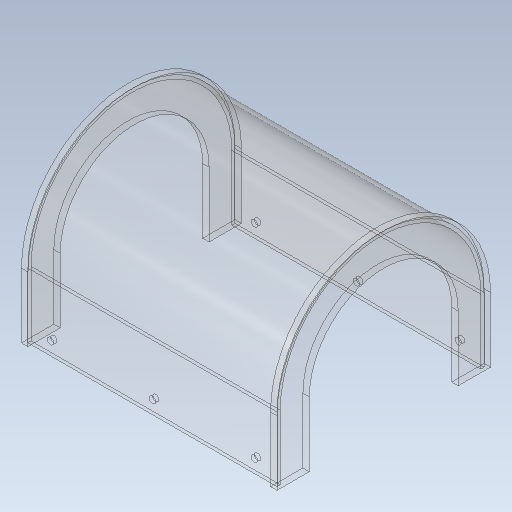
# Autodesk Inventor part: Acrilico
Saved by Autodesk Inventor 2020 (Build 240168000, 168)
## iProperties
Created: 2018-06-05
Part Number: Acrilico
Material: Plástico PMMA
Document SubType Name: Chapa
Designer: Cristiano
Density: 1.188 g/cm^3
Appearance: Policarbonato - Claro
Mass: 1478.37 g
Surface Area: 5090.38 cm^2
Volume: 1244.42 cm^3
Sheet Metal Rule: Por defecto_mm
Sheet Metal Width: 0,000 mm
Sheet Metal Length: 0,000 mm
Sheet Metal Area: 0,000 mm^2
Author: Cristiano
Autodesk Inventor part; units mm, degrees
ref_plane "YZ Plane" through (0, 0, 0) normal (1, 0, 0) x (0, 1, 0)
ref_plane "XZ Plane" through (0, 0, 0) normal (0, 1, 0) x (-1, 0, 0)
ref_plane "XY Plane" through (0, 0, 0) normal (0, 0, 1) x (1, 0, 0)
sketch "Boceto1" plane through (0, 0, 0) normal (1, 0, 0) x (0, 1, 0)
  line L0 (0, 0) -> (0, -220.3761) construction
  arc A0 (0, -155) -> (0, 155) centre (0, 0) ccw
  arc A1 (0, -160) -> (0, 160) centre (0, 0) ccw
  line L1 (0, 155) -> (0, 160) construction
  line L2 (0, -155) -> (0, -160) construction
  line L3 (0, -160) -> (-100, -160)
  line L4 (-100, -160) -> (-100, -155)
  line L5 (-100, -155) -> (0, -155)
  line L6 (0, 155) -> (-100, 155)
  line L7 (-100, 155) -> (-100, 160)
  line L8 (0, 160) -> (-100, 160)
  dimension "d1" = 155
  dimension "d4" = 160
  dimension "d7" = 100
  dimension "d8" = 5
  constraints: 18 end point, 4 point on circle, 3 collinear, 3 horizontal, 3 vertical, 2 centre point, 2 perpendicular, 1 coincident
  measures "d1" radius of A0
  measures "d4" radius of A1
  measures "d7" distance of L2.end L3.end
  measures "d8" distance of L6.end L7.end
extrude "Extrusión1" add sketch "Boceto1" along normal blind 385
sketch "Boceto2" plane through (0, -100, -160) normal (0, 0, -1) x (-1, 0, 0)
  line L0 (-385, 0) -> (-385, 100) construction
  line L1 (-385, 20) -> (0, 20) construction
  line L2 (0, 0) -> (0, 100) construction
  circle A0 centre (-350, 20) radius 5
  circle A1 centre (-192.5, 20) radius 5
  circle A2 centre (-35, 20) radius 5
  dimension "d9" = 10
  dimension "d10" = 35
  dimension "d11" = 35
  dimension "d14" = 20
  constraints: 4 point on line, 3 centre point, 2 end point, 2 equal radius, 1 midpoint, 1 perpendicular
  measures "d9" diameter of A0
  measures "d10" distance from line of L0 A0.centre
  measures "d11" distance from line of L2 A2.centre
  measures "d14" distance of L0.start L1.start
extrude "Extrusión2" cut sketch "Boceto2" against normal through all
ref_plane "Plano de trabajo1" through (192.5, 0, 0) normal (1, 0, 0) x (0, 0, -1)
sketch "Boceto3" plane through (385, 0, 0) normal (1, 0, 0) x (0, 0, -1)
  line L0 (-160, 0) -> (-160, -100) construction
  arc A0 (160, 0) -> (-160, 0) centre (0, 0) ccw construction
  line L1 (160, -100) -> (160, 0) construction
  line L2 (-165, -100) -> (-165, 0)
  arc A1 (165, 0) -> (-165, 0) centre (0, 0) ccw
  line L3 (165, 0) -> (165, -100)
  line L4 (-115, -100) -> (-115, 0)
  arc A2 (115, 0) -> (-115, 0) centre (0, 0) ccw
  line L5 (115, 0) -> (115, -100)
  line L6 (-165, -100) -> (-115, -100)
  line L7 (115, -100) -> (165, -100)
  line L8 (155, -100) -> (160, -100) projected
  line L9 (-160, -100) -> (-155, -100) projected
  dimension "d15" = 5
  dimension "d19" = 50
  constraints: 12 end point, 4 point on circle, 3 collinear, 2 centre point, 1 horizontal, 4 other
  measures "d15" radial gap between concentric circles of A0 A1
  measures "d19" distance of L5.end L3.end
extrude "Extrusión3" add sketch "Boceto3" along normal mid plane 10 separate body
mirror "Simetría1" about plane through (192.5, 0, 0) normal (1, 0, 0) of "Extrusión3" bodies 2
ref_plane "Plano de trabajo2" through (192.5, 0, 0) normal (1, 0, 0) x (0, 0, -1)
equation "\"Radio_pliegue\" = Grosor"
equation "\"Anchura_desahogo_plegado\" = Grosor"
equation "\"Profundidad_desahogo_plegado\" = 0.5 * Grosor"
equation "\"Radiodetransición\" = Radio_pliegue"
equation "\"Tamaño_de_radio_de_Jacobi\" = Radio_pliegue"
equation "\"TamañoSeparación\" = Grosor"
equation "\"Grosor\" = 5"
